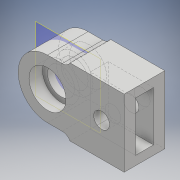
# Autodesk Inventor part: center-machine-v2-rod-socket
Saved by Autodesk Inventor 2018 (Build 220112000, 112)
## iProperties
Created: 2025-09-19
Part Number: center-machine-v2-rod-socket
Material: Generic
Document SubType Name: Modeling
Designer: neo
Density: 1 g/cm^3
Appearance: Default
Author: neo
Autodesk Inventor part; units mm, degrees
ref_plane "YZ Plane" through (0, 0, 0) normal (1, 0, 0) x (0, 1, 0)
ref_plane "XZ Plane" through (0, 0, 0) normal (0, 1, 0) x (-1, 0, 0)
ref_plane "XY Plane" through (0, 0, 0) normal (0, 0, 1) x (1, 0, 0)
sketch "Sketch1" plane through (0, 0, 0) normal (0, 1, 0) x (-1, 0, 0)
  circle A0 centre (0, 0) radius 2
  circle A1 centre (0, 0) radius 4 construction
  circle A2 centre (0, 0) radius 6.5
  dimension "d0" = 4
  dimension "d1" = 8
  dimension "d2" = 13
  constraints: 3 centre point, 3 coincident
  measures "d0" diameter of A0
  measures "d1" diameter of A1
  measures "d2" diameter of A2
extrude "Extrusion1" add sketch "Sketch1" against normal blind 9
ref_plane "Work Plane1" through (0, -4.5, 0) normal (0, 1, 0) x (1, 0, 0)
hole "Hole1" at (0, 0, 0) direction (0, -1, 0) diameter 6 end through all counterbore diameter 8.2 counterbore depth 3
mirror "Mirror1" about plane through (0, -4.5, 0) normal (0, 1, 0) of "Hole1"
sketch "Sketch2" plane through (0, -4.5, 0) normal (0, 1, 0) x (1, 0, 0)
  circle A0 centre (0, 0) radius 4.1 projected
  circle A1 centre (0, 0) radius 6.5 projected
  line L0 (0, -6.5) -> (16.9987, -6.5)
  line L1 (16.9987, -6.5) -> (16.9987, 6.5)
  line L2 (16.9987, 6.5) -> (-0.0013, 6.5)
  arc A2 (-0.0013, 6.5) -> (0, -6.5) centre (0, 0) ccw
  dimension "d14" = 17
  constraints: 6 end point, 2 point on circle, 1 centre point, 1 horizontal, 1 parallel, 1 perpendicular, 1 tangent, 1 vertical alignment, 1 other
  measures "d14" distance of L1.end L2.end
extrude "Extrusion2" add sketch "Sketch2" against normal up to surface (9 mm away) from surface at 4.5 contours A1 L2 L1 L0
sketch "Sketch3" plane through (16.9987, -9, -6.5) normal (1, 0, 0) x (0, 0, -1)
  line L0 (-13, 0) -> (-13, 9) construction
  line L1 (-13, 4.5) -> (0, 4.5) construction
  line L2 (0, 0) -> (0, 9) construction
  line L3 (-6.5, 9) -> (-6.5, -1) construction
  line L4 (-12, 6.5) -> (-1, 6.5)
  line L5 (-1, 6.5) -> (-1, 2.5)
  line L6 (-1, 2.5) -> (-12, 2.5)
  line L7 (-12, 2.5) -> (-12, 6.5)
  dimension "d17" = 11
  dimension "d18" = 4
  constraints: 12 end point, 2 midpoint, 2 parallel, 1 horizontal, 1 perpendicular, 1 vertical, 2 other
  measures "d17" distance between parallel lines of L7 L5
  measures "d18" distance between parallel lines of L6 L4
extrude "Extrusion3" cut sketch "Sketch3" against normal blind 10
sketch "Sketch4" plane through (0, -4.5, 0) normal (0, 1, 0) x (1, 0, 0)
  line L0 (16.9987, 6.5) -> (16.9987, -6.5) projected
  line L1 (16.9987, -6.5) -> (4.9987, -6.5)
  line L2 (4.9987, -6.5) -> (4.9987, -7.5)
  line L3 (4.9987, -7.5) -> (16.9987, -7.5)
  line L4 (16.9987, -7.5) -> (16.9987, -6.5)
  line L5 (0, 0) -> (21.5191, 0) construction
  line L6 (16.9987, 6.5) -> (4.9987, 6.5)
  line L7 (4.9987, 6.5) -> (4.9987, 7.5)
  line L8 (4.9987, 7.5) -> (16.9987, 7.5)
  line L9 (16.9987, 7.5) -> (16.9987, 6.5)
  dimension "d21" = 1
  dimension "d22" = 12
  constraints: 18 end point, 3 symmetric about line, 2 horizontal, 2 parallel, 1 perpendicular
  measures "d21" distance of L3.end L0.end
  measures "d22" distance of L2.end L3.end
extrude "Extrusion4" add sketch "Sketch4" against normal up to surface (9 mm away) from surface at 4.5
fillet "Fillet1" radius 2 2 edges at (4.9987, -4.5, -6.5) (4.9987, -4.5, 6.5)
sketch "Sketch5" plane through (0, -4.5, 0) normal (0, 1, 0) x (1, 0, 0)
  line L0 (16.9987, -5.5) -> (6.9987, -5.5) construction
  line L1 (6.9987, -5.5) -> (6.9987, 5.5) construction
  line L2 (16.9987, 5.5) -> (6.9987, 5.5) construction
  line L3 (6.9987, 0) -> (20.6867, 0) construction
  line L4 (11.9987, -5.5) -> (11.9987, 4.4002) construction
  circle A0 centre (11.9987, 0) radius 1.75
  point P0 (0, 0)
  dimension "d26" = 3.5
  constraints: 4 end point, 2 midpoint, 2 point on line, 1 centre point, 1 horizontal, 1 vertical
  measures "d26" diameter of A0
extrude "Extrusion5" cut sketch "Sketch5" along normal through all both and the other way through all
body "Solid1"
